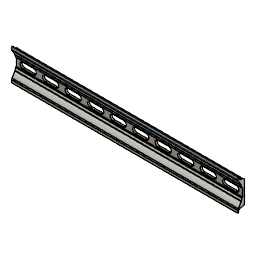
Printable+Din+Rail+v2 v1 (Autodesk Fusion 360 design; units mm, degrees)
description: STEP AP203
Autodesk Fusion 360 part; units mm, degrees
imported_body "Base Feature1" makes body 1 makes body 2
sketch "Sketch1" plane through (0, 0, 0) normal (1, 0, 0) x (0, 0, -1)
  arc A0 (-7.021, -13.2013) -> (-7.5, -14.5) centre (-5.5, -14.5) ccw
  line L0 (-7.5, -14.5) -> (-7.5, -17.5)
  line L1 (-7.5, -17.5) -> (-6.5, -17.5)
  line L2 (-6.5, -17.5) -> (-6.5, -16.5)
  arc A1 (-3.5, -13.5) -> (-6.5, -16.5) centre (-3.5, -16.5) ccw
  line L3 (-3.5, -13.5) -> (-2, -13.5)
  arc A2 (-2, -13.5) -> (0, -11.5) centre (-2, -11.5) ccw
  line L4 (0, -11.5) -> (0, 11.5)
  arc A3 (0, 11.5) -> (-2, 13.5) centre (-2, 11.5) ccw
  line L5 (-2, 13.5) -> (-3.5, 13.5)
  arc A4 (-6.5, 16.5) -> (-3.5, 13.5) centre (-3.5, 16.5) ccw
  line L6 (-6.5, 16.5) -> (-6.5, 17.5)
  line L7 (-6.5, 17.5) -> (-7.5, 17.5)
  line L8 (-7.5, 17.5) -> (-7.5, 14.5)
  arc A5 (-7.5, 14.5) -> (-7.021, 13.2013) centre (-5.5, 14.5) ccw
  arc A6 (-3.7416, 7.6132) -> (-7.021, 13.2013) centre (-21.0901, 1.1884) ccw
  arc A7 (-3.7416, 7.6132) -> (-3.8046, 7.7905) centre (-25.445, 0) ccw
  line L9 (-3.8046, 7.7905) -> (-3.6837, 7.4547)
  arc A8 (-3.6837, 7.4547) -> (-3.7416, 7.6132) centre (-21.0901, 1.1884) ccw
  arc A9 (-2.9716, 4.8936) -> (-3.7416, 7.6132) centre (-25.445, 0) ccw
  arc A10 (-2.9716, 4.8936) -> (-2.4831, 4.5) centre (-2.4831, 5) ccw
  line L10 (-2.4831, 4.5) -> (-2.1215, 4.5)
  line L11 (-2.1215, 4.5) -> (-2.1215, -4.5)
  line L12 (-2.1215, -4.5) -> (-2.4831, -4.5)
  arc A11 (-2.4831, -4.5) -> (-2.9716, -4.8936) centre (-2.4831, -5) ccw
  arc A12 (-3.7416, -7.6132) -> (-2.9716, -4.8936) centre (-25.445, 0) ccw
  arc A13 (-3.7416, -7.6132) -> (-3.6837, -7.4547) centre (-21.0901, -1.1884) ccw
  line L13 (-3.6837, -7.4547) -> (-3.8046, -7.7905)
  arc A14 (-3.8046, -7.7905) -> (-3.7416, -7.6132) centre (-25.445, 0) ccw
  arc A15 (-7.021, -13.2013) -> (-3.7416, -7.6132) centre (-21.0901, -1.1884) ccw
sketch "Sketch2" plane through (0, 0, 0) normal (0, 0, -1) x (1, 0, 0)
  arc A0 (-244, 3.15) -> (-245, 2.9871) centre (-244, 0) ccw
  line L0 (-244, 3.15) -> (-232.3, 3.15)
  arc A1 (-232.2999, -3.15) -> (-232.3, 3.15) centre (-232.3, 0) ccw
  line L1 (-232.2999, -3.15) -> (-244, -3.15)
  arc A2 (-245, -2.9871) -> (-244, -3.15) centre (-244, 0) ccw
  line L2 (-245, -2.9871) -> (-245, -11.5)
  line L3 (-245, -11.5) -> (0, -11.5)
  line L4 (0, -11.5) -> (0, 11.5)
  line L5 (0, 11.5) -> (-245, 11.5)
  line L6 (-245, 11.5) -> (-245, 2.9871)
  line L7 (-132.2999, -3.15) -> (-144, -3.15)
  arc A3 (-144, 3.15) -> (-144, -3.15) centre (-144, 0) ccw
  line L8 (-144, 3.15) -> (-132.3, 3.15)
  arc A4 (-132.2999, -3.15) -> (-132.3, 3.15) centre (-132.3, 0) ccw
  line L9 (-44, 3.15) -> (-32.3, 3.15)
  arc A5 (-32.2999, -3.15) -> (-32.3, 3.15) centre (-32.3, 0) ccw
  line L10 (-32.2999, -3.15) -> (-44, -3.15)
  arc A6 (-44, 3.15) -> (-44, -3.15) centre (-44, 0) ccw
  line L11 (-69, 3.15) -> (-57.3, 3.15)
  arc A7 (-57.2999, -3.15) -> (-57.3, 3.15) centre (-57.3, 0) ccw
  line L12 (-57.2999, -3.15) -> (-69, -3.15)
  arc A8 (-69, 3.15) -> (-69, -3.15) centre (-69, 0) ccw
  line L13 (-169, 3.15) -> (-157.3, 3.15)
  arc A9 (-157.2999, -3.15) -> (-157.3, 3.15) centre (-157.3, 0) ccw
  line L14 (-157.2999, -3.15) -> (-169, -3.15)
  arc A10 (-169, 3.15) -> (-169, -3.15) centre (-169, 0) ccw
  line L15 (-207.2999, -3.15) -> (-219, -3.15)
  arc A11 (-219, 3.15) -> (-219, -3.15) centre (-219, 0) ccw
  line L16 (-219, 3.15) -> (-207.3, 3.15)
  arc A12 (-207.2999, -3.15) -> (-207.3, 3.15) centre (-207.3, 0) ccw
  line L17 (-107.2999, -3.15) -> (-119, -3.15)
  arc A13 (-119, 3.15) -> (-119, -3.15) centre (-119, 0) ccw
  line L18 (-119, 3.15) -> (-107.3, 3.15)
  arc A14 (-107.2999, -3.15) -> (-107.3, 3.15) centre (-107.3, 0) ccw
  line L19 (-19, 3.15) -> (-7.3, 3.15)
  arc A15 (-7.2999, -3.15) -> (-7.3, 3.15) centre (-7.3, 0) ccw
  line L20 (-7.2999, -3.15) -> (-19, -3.15)
  arc A16 (-19, 3.15) -> (-19, -3.15) centre (-19, 0) ccw
  line L21 (-94, 3.15) -> (-82.3, 3.15)
  arc A17 (-82.2999, -3.15) -> (-82.3, 3.15) centre (-82.3, 0) ccw
  line L22 (-82.2999, -3.15) -> (-94, -3.15)
  arc A18 (-94, 3.15) -> (-94, -3.15) centre (-94, 0) ccw
  line L23 (-182.2999, -3.15) -> (-194, -3.15)
  arc A19 (-194, 3.15) -> (-194, -3.15) centre (-194, 0) ccw
  line L24 (-194, 3.15) -> (-182.3, 3.15)
  arc A20 (-182.2999, -3.15) -> (-182.3, 3.15) centre (-182.3, 0) ccw
  arc A21 (-244, 3.15) -> (-244, -3.15) centre (-244, 0) ccw
  line L25 (-244, 0) -> (-251.3, 0)
  line L26 (-251.3, 0) -> (0, 0)
  dimension "d1" = 7.3
  constraint coincident A0.centre A2.centre
  constraint perpendicular L6 L25
  constraint coincident L26.end origin
  measures "d1" distance of A0.centre L25.end
extrude "Extrude1" add sketch "Sketch1" against normal blind 251.3 separate body makes body 3
sketch "sketch 1749" plane through (0, 0, 0) normal (0, 0, -1) x (-1, 0, 0)
  line L0 (0, 11.5) -> (0, -11.5)
  line L1 (0, -11.5) -> (245, -11.5)
  line L2 (245, -11.5) -> (245, 11.5)
  line L3 (245, 11.5) -> (0, 11.5)
  line L4 (0, 0) -> (245, 0) construction
  line L5 (0, 0) -> (24.5, 0) construction
  line L6 (12.25, 0) -> (12.25, 11.5) construction
  line L7 (0, -11.5) -> (100, -11.5)
  line L8 (100, -11.5) -> (100, 11.5)
  line L9 (100, 11.5) -> (0, 11.5)
  line L10 (0, 11.5) -> (0, -11.5)
  line L11 (69, -3.15) -> (57.3, -3.15)
  arc A0 (57.2999, 3.15) -> (57.3, -3.15) centre (57.3, 0) ccw
  line L12 (57.2999, 3.15) -> (69, 3.15)
  arc A1 (69, -3.15) -> (69, 3.15) centre (69, 0) ccw
  line L13 (44, -3.15) -> (32.3, -3.15)
  arc A2 (32.2999, 3.15) -> (32.3, -3.15) centre (32.3, 0) ccw
  line L14 (32.2999, 3.15) -> (44, 3.15)
  arc A3 (44, -3.15) -> (44, 3.15) centre (44, 0) ccw
  line L15 (19, -3.15) -> (7.3, -3.15)
  arc A4 (7.2999, 3.15) -> (7.3, -3.15) centre (7.3, 0) ccw
  line L16 (7.2999, 3.15) -> (19, 3.15)
  arc A5 (19, -3.15) -> (19, 3.15) centre (19, 0) ccw
  arc A6 (94, -3.15) -> (94, 3.15) centre (94, 0) ccw
  line L17 (94, -3.15) -> (82.3, -3.15)
  arc A7 (82.2999, 3.15) -> (82.3, -3.15) centre (82.3, 0) ccw
  line L18 (82.2999, 3.15) -> (94, 3.15)
  line L19 (144, -3.15) -> (132.3, -3.15)
  line L20 (107.2999, 3.15) -> (119, 3.15)
  line L21 (94, -3.15) -> (82.3, -3.15)
  arc A8 (169, -3.15) -> (169, 3.15) centre (169, 0) ccw
  line L22 (82.2999, 3.15) -> (94, 3.15)
  arc A9 (119, -3.15) -> (119, 3.15) centre (119, 0) ccw
  arc A10 (132.2999, 3.15) -> (132.3, -3.15) centre (132.3, 0) ccw
  line L23 (169, -3.15) -> (157.3, -3.15)
  line L24 (157.2999, 3.15) -> (169, 3.15)
  arc A11 (144, -3.15) -> (144, 3.15) centre (144, 0) ccw
  arc A12 (157.2999, 3.15) -> (157.3, -3.15) centre (157.3, 0) ccw
  line L25 (119, -3.15) -> (107.3, -3.15)
  arc A13 (82.2999, 3.15) -> (82.3, -3.15) centre (82.3, 0) ccw
  line L26 (132.2999, 3.15) -> (144, 3.15)
  arc A14 (107.2999, 3.15) -> (107.3, -3.15) centre (107.3, 0) ccw
  arc A15 (94, -3.15) -> (94, 3.15) centre (94, 0) ccw
  line L27 (219, -3.15) -> (207.3, -3.15)
  line L28 (182.2999, 3.15) -> (194, 3.15)
  line L29 (169, -3.15) -> (157.3, -3.15)
  arc A16 (244, -3.15) -> (244, 3.15) centre (244, 0) ccw
  line L30 (157.2999, 3.15) -> (169, 3.15)
  arc A17 (194, -3.15) -> (194, 3.15) centre (194, 0) ccw
  arc A18 (207.2999, 3.15) -> (207.3, -3.15) centre (207.3, 0) ccw
  line L31 (244, -3.15) -> (232.3, -3.15)
  line L32 (232.2999, 3.15) -> (244, 3.15)
  arc A19 (219, -3.15) -> (219, 3.15) centre (219, 0) ccw
  arc A20 (232.2999, 3.15) -> (232.3, -3.15) centre (232.3, 0) ccw
  line L33 (194, -3.15) -> (182.3, -3.15)
  arc A21 (157.2999, 3.15) -> (157.3, -3.15) centre (157.3, 0) ccw
  line L34 (207.2999, 3.15) -> (219, 3.15)
  arc A22 (182.2999, 3.15) -> (182.3, -3.15) centre (182.3, 0) ccw
  arc A23 (169, -3.15) -> (169, 3.15) centre (169, 0) ccw
  constraint coincident L4.start L5.start
  constraint midpoint L2 L4.end
  constraint perpendicular L2 L5
  constraint midpoint L5 L6.start
  constraint coincident L3 L6.end
  constraint perpendicular L3 L6
extrude "Extrude2" cut sketch "Sketch2" sketch "sketch 1749" against normal blind 20 contours L19 A15 A16 L26 | A15 L20 A16 L26 | L17 A13 A14 L26 of sketch 2 contours L2 A16 | L2 A16 L31 L32 A20 | L11 A0 L12 A1 | L13 A2 L14 A3 | A6 L17 A7 L18 L21 L22 A13 A15 | L19 A10 A11 L26 | L20 A9 L25 A14 | A8 L23 L24 A12 L29 L30 A21 A23 | L27 A18 A19 L34 | L28 A17 L33 A22 bodies 3
sketch "Sketch3" plane through (0, 0, 7.5) normal (0, 0, 1) x (1, 0, 0)
  line L0 (0, 14.5) -> (0, 17.5)
  line L1 (0, 17.5) -> (-251.3, 17.5)
  line L2 (-251.3, 17.5) -> (-251.3, 14.5)
  line L3 (-251.3, 14.5) -> (0, 14.5)
hidden bodies 1 2
named bodies: "251.3mm DIn Rail"
